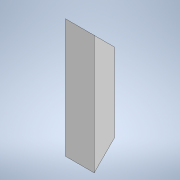
# Autodesk Inventor part: Middle
Saved by Autodesk Inventor 2020 (Build 240168000, 168)
## iProperties
Created: 2020-11-08
Part Number: Middle
Material: Generic
Document SubType Name: Modeling
Designer: user
Density: 1 g/cm^3
Appearance: Default
Author: user
Autodesk Inventor part; units mm, degrees
ref_plane "YZ Plane" through (0, 0, 0) normal (1, 0, 0) x (0, 1, 0)
ref_plane "XZ Plane" through (0, 0, 0) normal (0, 1, 0) x (-1, 0, 0)
ref_plane "XY Plane" through (0, 0, 0) normal (0, 0, 1) x (1, 0, 0)
sketch "Sketch1" plane through (0, 0, 0) normal (0, 1, 0) x (-1, 0, 0)
  line L0 (4.7038, 2.0376) -> (-7.2962, 2.0376)
  line L1 (-7.2962, 2.0376) -> (-7.2962, -6.4474)
  line L2 (-7.2962, -6.4474) -> (4.7038, -6.4474)
  line L3 (4.7038, -6.4474) -> (4.7038, 2.0376)
  point P0 (0, 0)
  dimension "d0" = 12
  dimension "d1" = 8.485
  constraints: 8 end point, 2 parallel, 1 horizontal, 1 perpendicular
  measures "d0" distance of L2.end L1.end
  measures "d1" distance of L1.end L0.end
extrude "Extrusion1" add sketch "Sketch1" along normal blind 50
sketch "Sketch5" plane through (7.2962, 0, 2.0376) normal (1, 0, 0) x (0, 0, -1)
  line L0 (0, 0) -> (0, 50) projected
  line L1 (0, 50) -> (8.485, 41.515)
  line L2 (8.485, 0) -> (8.485, 50) projected
  line L3 (0, 50) -> (8.485, 50) projected
  line L4 (0, 0) -> (8.485, 0) projected
  line L5 (0, 0) -> (8.485, 8.485)
  point P0 (2.0376, 0)
  dimension "d11" = 45
  dimension "d15" = 45
  constraints: 4 end point, 2 point on line
  measures "d11" angle of L1 L3
  measures "d15" angle of L4 L5
extrude "Extrusion4" cut sketch "Sketch5" against normal blind 12 contours L5 L2 L4 | L3 L2 L1
body "Solid1"
